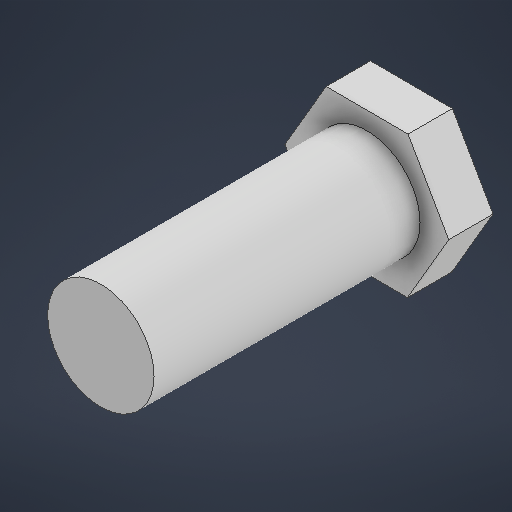
# Autodesk Inventor part: nut2
Saved by Autodesk Inventor 2026 (Build 300175000, 175)
## iProperties
Created: 2025-05-08
Part Number: nut2
Material: Generic
Document SubType Name: Modeling
Designer: Ritul Kumari
Density: 1 g/cm^3
Appearance: Default
Author: Ritul Kumari
Autodesk Inventor part; units mm, degrees
ref_plane "YZ Plane" through (0, 0, 0) normal (1, 0, 0) x (0, 1, 0)
ref_plane "XZ Plane" through (0, 0, 0) normal (0, 1, 0) x (-1, 0, 0)
ref_plane "XY Plane" through (0, 0, 0) normal (0, 0, 1) x (1, 0, 0)
sketch "Sketch1" plane through (0, 0, 0) normal (0, 0, 1) x (1, 0, 0)
  point P0 (0, 0)
sketch "Sketch2" plane through (0, 0, 0) normal (0, 0, 1) x (1, 0, 0)
  line L0 (118.1199, 202.7368) -> (234.6351, -0.9265)
  line L1 (234.6351, -0.9265) -> (116.5152, -203.6632)
  line L2 (116.5152, -203.6632) -> (-118.1199, -202.7368)
  line L3 (-118.1199, -202.7368) -> (-234.6351, 0.9265)
  line L4 (-234.6351, 0.9265) -> (-116.5152, 203.6632)
  line L5 (-116.5152, 203.6632) -> (118.1199, 202.7368)
  point P0 (0, 0)
  point P1 (0, 0)
  point P2 (-0.8024, -203.2)
  point P3 (0.8024, 203.2)
  dimension "d0" = 406.4
  constraints: 12 end point, 2 midpoint, 1 coincident, 13 other
  measures "d0" vertical distance of point (-0.802, -203.2) point (0.802, 203.2)
extrude "Extrusion1" add sketch "Sketch2" along normal blind 127
sketch "Sketch3" plane through (0, 0, 127) normal (0, 0, 1) x (1, 0, 0)
  circle A0 centre (0, 0) radius 152.4
  dimension "d3" = 304.8
  constraints: 1 centre point, 1 coincident
  measures "d3" diameter of A0
extrude "Extrusion2" add sketch "Sketch3" along normal blind 762
body "Solid1"
